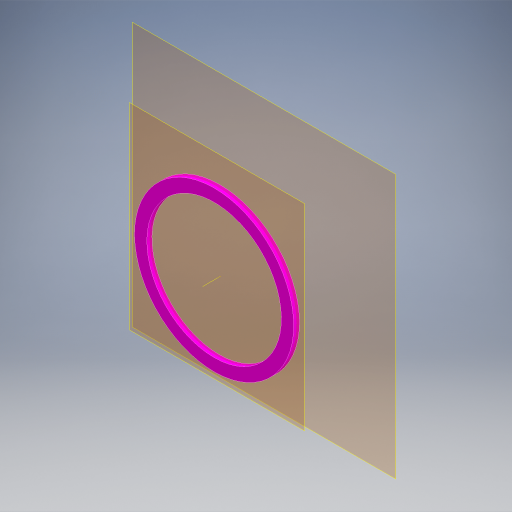
# Autodesk Inventor part: кольцо тсопов
Saved by Autodesk Inventor 2023 (Build 270158000, 158)
## iProperties
Created: 2025-03-03
Part Number: кольцо тсопов
Material: Типовые
Document SubType Name: Modeling
Designer: Ivan
Density: 1 g/cm^3
Appearance: Пурпурный
Author: Ivan
Autodesk Inventor part; units mm, degrees
ref_plane "YZ Plane" through (0, 0, 0) normal (1, 0, 0) x (0, 1, 0)
ref_plane "XZ Plane" through (0, 0, 0) normal (0, 1, 0) x (-1, 0, 0)
ref_plane "РабПлоскость1" through (0, 0, 0) normal (0, 0, 1) x (1, 0, 0)
sketch "Эскиз1" plane through (0, 0, 0) normal (0, 0, 1) x (1, 0, 0)
  circle A0 centre (-0.0031, 0.0005) radius 45.313 projected
  arc A1 (-32.0981, 35.7243) -> (-32.4617, 35.3942) centre (0, 0) ccw projected
  circle A2 centre (0, 0) radius 45.413
  circle A3 centre (0, 0) radius 48.0262
  point P0 (0, 0)
  point P1 (-32.4617, 35.3942)
  point P2 (-32.0981, 35.7243)
  dimension "d0" = 90.626
  dimension "d1" = 90.826
  constraints: 2 centre point, 2 coincident
  measures "d0" diameter of A0
  measures "d1" diameter of A2
ref_plane "РабПлоскость2" through (-45.3206, -45.317, 0.4115) normal (0, 0, 1) x (1, 0.0001, 0)
extrude "Выдавливание1" add sketch "Эскиз1" along normal blind 3.5 contours A3 A1
ref_plane "РабПлоскость3" through (0, 0, 1.75) normal (0, 0, 1) x (1, 0, 0)
sketch "Эскиз3" plane through (0, 0, 0) normal (0, 0, 1) x (1, 0, 0)
  arc A0 (-22.0856, 39.6831) -> (-7.3436, 35.1497) centre (-7.7664, 60.011) ccw projected
  line L0 (-7.3436, 35.1497) -> (7.3325, 35.1512) projected
  arc A1 (7.3325, 35.1512) -> (22.0736, 39.6875) centre (7.7504, 60.0125) ccw projected
  circle A2 centre (0, 0) radius 45.413 projected
  circle A3 centre (-15.1051, 31) radius 1.55 projected
  circle A4 centre (15.0949, 31.002) radius 1.55 projected
  arc A5 (-17.5837, 28.9218) -> (-32.0889, 32.1347) centre (-28.1894, 15.3907) ccw projected
  arc A6 (-16.8937, 28.4734) -> (-17.5837, 28.9218) centre (-22.6832, 20.3197) ccw projected
  arc A7 (-16.8937, 28.4734) -> (-9.3575, 28.0766) centre (-12.8523, 33.4648) ccw projected
  arc A8 (-5.0551, 30.151) -> (-5.054, 19.151) centre (-5.0545, 24.651) ccw projected
  line L1 (5.0449, 30.151) -> (-5.0551, 30.151) projected
  arc A9 (5.046, 19.151) -> (5.0449, 30.151) centre (5.0455, 24.651) ccw projected
  arc A10 (9.3461, 28.0795) -> (16.884, 28.4767) centre (12.8416, 33.4673) ccw projected
  arc A11 (17.5738, 28.9252) -> (16.884, 28.4767) centre (22.675, 20.3242) ccw projected
  arc A12 (32.0838, 32.1398) -> (17.5738, 28.9252) centre (28.1822, 15.3963) ccw projected
  point P0 (0, 0)
  point P1 (-22.0837, 39.6818)
extrude "Выдавливание2" [suppressed]
sketch "Эскиз4" plane through (0, 0, 0) normal (0, 0, -1) x (-1, 0, 0)
  circle A0 centre (-15.099, -31.001) radius 1.6 projected
  circle A1 centre (15.101, -31) radius 1.6 projected
  circle A2 centre (-15.101, 31) radius 1.6 projected
  circle A3 centre (15.099, 31.001) radius 1.6 projected
  arc A4 (47.464, 7.3269) -> (46.1696, 9.1429) centre (45.0118, 6.9484) ccw projected
  line L0 (46.1696, 9.1429) -> (46.154, 9.2214) projected
  arc A5 (46.154, 9.2214) -> (46.6549, 11.3945) centre (44.2445, 10.8058) ccw projected
  arc A6 (46.6549, 11.3945) -> (46.5359, 11.8709) centre (0, 0) ccw projected
  arc A7 (45.1226, 16.4459) -> (43.4988, 17.9745) centre (42.7913, 15.5962) ccw projected
  line L1 (43.4988, 17.9745) -> (43.4682, 18.0484) projected
  arc A8 (43.4682, 18.0484) -> (43.5355, 20.2775) centre (41.2862, 19.2298) ccw projected
  arc A9 (43.5355, 20.2775) -> (43.3259, 20.7215) centre (0, 0) ccw projected
  arc A10 (41.0471, 24.9329) -> (39.1563, 26.1153) centre (38.9264, 23.6447) ccw projected
  line L2 (39.1563, 26.1153) -> (39.1119, 26.1818) projected
  arc A11 (39.1119, 26.1818) -> (38.743, 28.3812) centre (36.7414, 26.9149) ccw projected
  arc A12 (38.743, 28.3812) -> (38.4508, 28.7758) centre (0, 0) ccw projected
  arc A13 (35.3942, 32.4617) -> (33.3091, 33.2525) centre (33.5656, 30.7846) ccw projected
  line L3 (33.3091, 33.2525) -> (33.2525, 33.3091) projected
  arc A14 (33.2525, 33.3091) -> (32.4617, 35.3942) centre (30.7846, 33.5656) ccw projected
  arc A15 (32.4617, 35.3942) -> (32.0981, 35.7243) centre (0, 0) ccw projected
  arc A16 (28.3812, 38.743) -> (26.1818, 39.1119) centre (26.9149, 36.7414) ccw projected
  line L4 (26.1818, 39.1119) -> (26.1153, 39.1563) projected
  arc A17 (26.1153, 39.1563) -> (24.9329, 41.0471) centre (23.6447, 38.9264) ccw projected
  arc A18 (24.9329, 41.0471) -> (24.5119, 41.2999) centre (0, 0) ccw projected
  arc A19 (20.2775, 43.5355) -> (18.0484, 43.4682) centre (19.2298, 41.2862) ccw projected
  line L5 (18.0484, 43.4682) -> (17.9745, 43.4988) projected
  arc A20 (17.9745, 43.4988) -> (16.4459, 45.1226) centre (15.5962, 42.7913) ccw projected
  arc A21 (16.4459, 45.1226) -> (15.9837, 45.2884) centre (0, 0) ccw projected
  arc A22 (11.3945, 46.6549) -> (9.2214, 46.154) centre (10.8058, 44.2445) ccw projected
  line L6 (9.2214, 46.154) -> (9.1429, 46.1696) projected
  arc A23 (9.1429, 46.1696) -> (7.3269, 47.464) centre (6.9484, 45.0118) ccw projected
  arc A24 (7.3269, 47.464) -> (6.8412, 47.5364) centre (0, 0) ccw projected
  arc A25 (2.0736, 47.9814) -> (0.04, 47.0662) centre (1.9665, 45.5024) ccw projected
  line L7 (0.04, 47.0662) -> (-0.04, 47.0662) projected
  arc A26 (-0.04, 47.0662) -> (-2.0736, 47.9814) centre (-1.9665, 45.5024) ccw projected
  arc A27 (-2.0736, 47.9814) -> (-2.5641, 47.9577) centre (0, 0) ccw projected
  arc A28 (-7.3269, 47.464) -> (-9.1429, 46.1696) centre (-6.9484, 45.0118) ccw projected
  line L8 (-9.1429, 46.1696) -> (-9.2214, 46.154) projected
  arc A29 (-9.2214, 46.154) -> (-11.3945, 46.6549) centre (-10.8058, 44.2445) ccw projected
  arc A30 (-11.3945, 46.6549) -> (-11.8709, 46.5359) centre (0, 0) ccw projected
  arc A31 (-16.4459, 45.1226) -> (-17.9745, 43.4988) centre (-15.5962, 42.7913) ccw projected
  line L9 (-17.9745, 43.4988) -> (-18.0484, 43.4682) projected
  arc A32 (-18.0484, 43.4682) -> (-20.2775, 43.5355) centre (-19.2298, 41.2862) ccw projected
  arc A33 (-20.2775, 43.5355) -> (-20.7215, 43.3259) centre (0, 0) ccw projected
  arc A34 (-24.9329, 41.0471) -> (-26.1153, 39.1563) centre (-23.6447, 38.9264) ccw projected
  line L10 (-26.1153, 39.1563) -> (-26.1818, 39.1119) projected
  arc A35 (-26.1818, 39.1119) -> (-28.3812, 38.743) centre (-26.9149, 36.7414) ccw projected
  arc A36 (-28.3812, 38.743) -> (-28.7758, 38.4508) centre (0, 0) ccw projected
  arc A37 (-32.4617, 35.3942) -> (-33.2525, 33.3091) centre (-30.7846, 33.5656) ccw projected
  line L11 (-33.2525, 33.3091) -> (-33.3091, 33.2525) projected
  arc A38 (-33.3091, 33.2525) -> (-35.3942, 32.4617) centre (-33.5656, 30.7846) ccw projected
  arc A39 (-35.3942, 32.4617) -> (-35.7243, 32.0981) centre (0, 0) ccw projected
  arc A40 (-38.743, 28.3812) -> (-39.1119, 26.1818) centre (-36.7414, 26.9149) ccw projected
  line L12 (-39.1119, 26.1818) -> (-39.1563, 26.1153) projected
  arc A41 (-39.1563, 26.1153) -> (-41.0471, 24.9329) centre (-38.9264, 23.6447) ccw projected
  arc A42 (-41.0471, 24.9329) -> (-41.2999, 24.5119) centre (0, 0) ccw projected
  arc A43 (-43.5355, 20.2775) -> (-43.4682, 18.0484) centre (-41.2862, 19.2298) ccw projected
  line L13 (-43.4682, 18.0484) -> (-43.4988, 17.9745) projected
  arc A44 (-43.4988, 17.9745) -> (-45.1226, 16.4459) centre (-42.7913, 15.5962) ccw projected
  arc A45 (-45.1226, 16.4459) -> (-45.2884, 15.9837) centre (0, 0) ccw projected
  arc A46 (-46.6549, 11.3945) -> (-46.154, 9.2214) centre (-44.2445, 10.8058) ccw projected
  line L14 (-46.154, 9.2214) -> (-46.1696, 9.1429) projected
  arc A47 (-46.1696, 9.1429) -> (-47.464, 7.3269) centre (-45.0118, 6.9484) ccw projected
  arc A48 (-47.464, 7.3269) -> (-47.5364, 6.8412) centre (0, 0) ccw projected
  arc A49 (-47.9814, 2.0736) -> (-47.0662, 0.04) centre (-45.5024, 1.9665) ccw projected
  line L15 (-47.0662, 0.04) -> (-47.0662, -0.04) projected
  arc A50 (-47.0662, -0.04) -> (-47.9814, -2.0736) centre (-45.5024, -1.9665) ccw projected
  arc A51 (-47.9814, -2.0736) -> (-47.9577, -2.5641) centre (0, 0) ccw projected
  arc A52 (-47.464, -7.3269) -> (-46.1696, -9.1429) centre (-45.0118, -6.9484) ccw projected
  line L16 (-46.1696, -9.1429) -> (-46.154, -9.2214) projected
  arc A53 (-46.154, -9.2214) -> (-46.6549, -11.3945) centre (-44.2445, -10.8058) ccw projected
  arc A54 (-46.6549, -11.3945) -> (-46.5359, -11.8709) centre (0, 0) ccw projected
  arc A55 (-45.1226, -16.4459) -> (-43.4988, -17.9745) centre (-42.7913, -15.5962) ccw projected
  line L17 (-43.4988, -17.9745) -> (-43.4682, -18.0484) projected
  arc A56 (-43.4682, -18.0484) -> (-43.5355, -20.2775) centre (-41.2862, -19.2298) ccw projected
  arc A57 (-43.5355, -20.2775) -> (-43.3259, -20.7215) centre (0, 0) ccw projected
  arc A58 (-41.0471, -24.9329) -> (-39.1563, -26.1153) centre (-38.9264, -23.6447) ccw projected
  line L18 (-39.1563, -26.1153) -> (-39.1119, -26.1818) projected
  arc A59 (-39.1119, -26.1818) -> (-38.743, -28.3812) centre (-36.7414, -26.9149) ccw projected
  arc A60 (-38.743, -28.3812) -> (-38.4508, -28.7758) centre (0, 0) ccw projected
  arc A61 (-35.3942, -32.4617) -> (-33.3091, -33.2525) centre (-33.5656, -30.7846) ccw projected
  line L19 (-33.3091, -33.2525) -> (-33.2525, -33.3091) projected
  arc A62 (-33.2525, -33.3091) -> (-32.4617, -35.3942) centre (-30.7846, -33.5656) ccw projected
  arc A63 (-32.4617, -35.3942) -> (-32.0981, -35.7243) centre (0, 0) ccw projected
  arc A64 (-28.3812, -38.743) -> (-26.1818, -39.1119) centre (-26.9149, -36.7414) ccw projected
  line L20 (-26.1818, -39.1119) -> (-26.1153, -39.1563) projected
  arc A65 (-26.1153, -39.1563) -> (-24.9329, -41.0471) centre (-23.6447, -38.9264) ccw projected
  arc A66 (-24.9329, -41.0471) -> (-24.5119, -41.2999) centre (0, 0) ccw projected
  arc A67 (-20.2775, -43.5355) -> (-18.0484, -43.4682) centre (-19.2298, -41.2862) ccw projected
  line L21 (-18.0484, -43.4682) -> (-17.9745, -43.4988) projected
  arc A68 (-17.9745, -43.4988) -> (-16.4459, -45.1226) centre (-15.5962, -42.7913) ccw projected
  arc A69 (-16.4459, -45.1226) -> (-15.9837, -45.2884) centre (0, 0) ccw projected
  arc A70 (-11.3945, -46.6549) -> (-9.2214, -46.154) centre (-10.8058, -44.2445) ccw projected
  line L22 (-9.2214, -46.154) -> (-9.1429, -46.1696) projected
  arc A71 (-9.1429, -46.1696) -> (-7.3269, -47.464) centre (-6.9484, -45.0118) ccw projected
  arc A72 (-7.3269, -47.464) -> (-6.8412, -47.5364) centre (0, 0) ccw projected
  arc A73 (-2.0736, -47.9814) -> (-0.04, -47.0662) centre (-1.9665, -45.5024) ccw projected
  line L23 (-0.04, -47.0662) -> (0.04, -47.0662) projected
  arc A74 (0.04, -47.0662) -> (2.0736, -47.9814) centre (1.9665, -45.5024) ccw projected
  arc A75 (2.0736, -47.9814) -> (2.5641, -47.9577) centre (0, 0) ccw projected
  arc A76 (7.3269, -47.464) -> (9.1429, -46.1696) centre (6.9484, -45.0118) ccw projected
  line L24 (9.1429, -46.1696) -> (9.2214, -46.154) projected
  arc A77 (9.2214, -46.154) -> (11.3945, -46.6549) centre (10.8058, -44.2445) ccw projected
  arc A78 (11.3945, -46.6549) -> (11.8709, -46.5359) centre (0, 0) ccw projected
  arc A79 (16.4459, -45.1226) -> (17.9745, -43.4988) centre (15.5962, -42.7913) ccw projected
  line L25 (17.9745, -43.4988) -> (18.0484, -43.4682) projected
  arc A80 (18.0484, -43.4682) -> (20.2775, -43.5355) centre (19.2298, -41.2862) ccw projected
  arc A81 (20.2775, -43.5355) -> (20.7215, -43.3259) centre (0, 0) ccw projected
  arc A82 (24.9329, -41.0471) -> (26.1153, -39.1563) centre (23.6447, -38.9264) ccw projected
  line L26 (26.1153, -39.1563) -> (26.1818, -39.1119) projected
  arc A83 (26.1818, -39.1119) -> (28.3812, -38.743) centre (26.9149, -36.7414) ccw projected
  arc A84 (28.3812, -38.743) -> (28.7758, -38.4508) centre (0, 0) ccw projected
  arc A85 (32.4617, -35.3942) -> (33.2525, -33.3091) centre (30.7846, -33.5656) ccw projected
  line L27 (33.2525, -33.3091) -> (33.3091, -33.2525) projected
  arc A86 (33.3091, -33.2525) -> (35.3942, -32.4617) centre (33.5656, -30.7846) ccw projected
  arc A87 (35.3942, -32.4617) -> (35.7243, -32.0981) centre (0, 0) ccw projected
  arc A88 (38.743, -28.3812) -> (39.1119, -26.1818) centre (36.7414, -26.9149) ccw projected
  line L28 (39.1119, -26.1818) -> (39.1563, -26.1153) projected
  arc A89 (39.1563, -26.1153) -> (41.0471, -24.9329) centre (38.9264, -23.6447) ccw projected
  arc A90 (41.0471, -24.9329) -> (41.2999, -24.5119) centre (0, 0) ccw projected
  arc A91 (43.5355, -20.2775) -> (43.4682, -18.0484) centre (41.2862, -19.2298) ccw projected
  line L29 (43.4682, -18.0484) -> (43.4988, -17.9745) projected
  arc A92 (43.4988, -17.9745) -> (45.1226, -16.4459) centre (42.7913, -15.5962) ccw projected
  arc A93 (45.1226, -16.4459) -> (45.2884, -15.9837) centre (0, 0) ccw projected
  arc A94 (46.6549, -11.3945) -> (46.154, -9.2214) centre (44.2445, -10.8058) ccw projected
  line L30 (46.154, -9.2214) -> (46.1696, -9.1429) projected
  arc A95 (46.1696, -9.1429) -> (47.464, -7.3269) centre (45.0118, -6.9484) ccw projected
  arc A96 (47.464, -7.3269) -> (47.5364, -6.8412) centre (0, 0) ccw projected
  arc A97 (47.9814, -2.0736) -> (47.0662, -0.04) centre (45.5024, -1.9665) ccw projected
  line L31 (47.0662, -0.04) -> (47.0662, 0.04) projected
  arc A98 (47.0662, 0.04) -> (47.9814, 2.0736) centre (45.5024, 1.9665) ccw projected
  arc A99 (47.9814, 2.0736) -> (47.9577, 2.5641) centre (0, 0) ccw projected
  arc A100 (27.9976, -29.0215) -> (27.9957, 29.0233) centre (0, 0) ccw projected
  arc A101 (22.6601, -30.3182) -> (27.9976, -29.0215) centre (22.6882, -18.8005) ccw projected
  arc A102 (16.8956, -28.4723) -> (22.6601, -30.3182) centre (22.6845, -20.3182) ccw projected
  arc A103 (16.8956, -28.4723) -> (12.0606, -31.6048) centre (15.101, -31) ccw projected
  arc A104 (5.6683, -39.9247) -> (12.0606, -31.6048) centre (4.6141, -32.4992) ccw projected
  arc A105 (-5.6658, -39.9251) -> (5.6683, -39.9247) centre (0, 0) ccw projected
  arc A106 (-12.0585, -31.6056) -> (-5.6658, -39.9251) centre (-4.612, -32.4995) ccw projected
  arc A107 (-12.0585, -31.6056) -> (-16.8937, -28.4734) centre (-15.099, -31.001) ccw projected
  arc A108 (-22.6581, -30.3197) -> (-16.8937, -28.4734) centre (-22.6832, -20.3197) ccw projected
  arc A109 (-27.9957, -29.0233) -> (-22.6581, -30.3197) centre (-22.687, -18.802) ccw projected
  arc A110 (-27.9976, 29.0215) -> (-27.9957, -29.0233) centre (0, 0) ccw projected
  arc A111 (-22.6601, 30.3182) -> (-27.9976, 29.0215) centre (-22.6882, 18.8005) ccw projected
  arc A112 (-16.8956, 28.4723) -> (-22.6601, 30.3182) centre (-22.6845, 20.3182) ccw projected
  arc A113 (-16.8956, 28.4723) -> (-12.0606, 31.6048) centre (-15.101, 31) ccw projected
  arc A114 (-5.6683, 39.9247) -> (-12.0606, 31.6048) centre (-4.6141, 32.4992) ccw projected
  arc A115 (5.6658, 39.9251) -> (-5.6683, 39.9247) centre (0, 0) ccw projected
  arc A116 (12.0585, 31.6056) -> (5.6658, 39.9251) centre (4.612, 32.4995) ccw projected
  arc A117 (12.0585, 31.6056) -> (16.8937, 28.4734) centre (15.099, 31.001) ccw projected
  arc A118 (22.6581, 30.3197) -> (16.8937, 28.4734) centre (22.6832, 20.3197) ccw projected
  arc A119 (27.9957, 29.0233) -> (22.6581, 30.3197) centre (22.687, 18.802) ccw projected
  circle A120 centre (0, 0) radius 48.0262 projected
  circle A121 centre (0, 0) radius 47.4785
  arc A122 (46.6623, -10.2485) -> (46.1696, -9.2404) centre (44.2445, -10.8058) ccw
  arc A123 (-3.4564, -47.5061) -> (-2.5641, -47.9577) centre (-2.4979, -46.7194) ccw projected
  arc A124 (-2.5641, -47.9577) -> (-2.0736, -47.9814) centre (0, 0) ccw projected
  arc A125 (2.5641, -47.9577) -> (3.4564, -47.5061) centre (2.4979, -46.7194) ccw projected
  line L32 (3.4564, -47.5061) -> (4.5479, -46.1761) projected
  line L33 (4.5479, -46.1761) -> (5.878, -47.2676) projected
  arc A126 (5.878, -47.2676) -> (6.8412, -47.5364) centre (6.6646, -46.3091) ccw projected
  arc A127 (6.8412, -47.5364) -> (7.3269, -47.464) centre (0, 0) ccw projected
  arc A128 (11.8709, -46.5359) -> (12.658, -45.9189) centre (11.5644, -45.3344) ccw projected
  line L34 (12.658, -45.9189) -> (13.4691, -44.4016) projected
  line L35 (13.4691, -44.4016) -> (14.9865, -45.2126) projected
  arc A129 (14.9865, -45.2126) -> (15.9837, -45.2884) centre (15.571, -44.119) ccw projected
  arc A130 (15.9837, -45.2884) -> (16.4459, -45.1226) centre (0, 0) ccw projected
  arc A131 (20.7215, -43.3259) -> (21.3731, -42.5672) centre (20.1865, -42.2072) ccw projected
  line L36 (21.3731, -42.5672) -> (21.8726, -40.9207) projected
  line L37 (21.8726, -40.9207) -> (23.519, -41.4202) projected
  arc A132 (23.519, -41.4202) -> (24.5119, -41.2999) centre (23.879, -40.2336) ccw projected
  arc A133 (24.5119, -41.2999) -> (24.9329, -41.0471) centre (0, 0) ccw projected
  arc A134 (28.7758, -38.4508) -> (29.2669, -37.5796) centre (28.0329, -37.458) ccw projected
  line L38 (29.2669, -37.5796) -> (29.4355, -35.8673) projected
  line L39 (29.4355, -35.8673) -> (31.1478, -36.0359) projected
  arc A135 (31.1478, -36.0359) -> (32.0981, -35.7243) centre (31.2693, -34.8019) ccw projected
  arc A136 (32.0981, -35.7243) -> (32.4617, -35.3942) centre (0, 0) ccw projected
  arc A137 (35.7243, -32.0981) -> (36.0359, -31.1478) centre (34.8019, -31.2693) ccw projected
  line L40 (36.0359, -31.1478) -> (35.8673, -29.4355) projected
  line L41 (35.8673, -29.4355) -> (37.5796, -29.2669) projected
  arc A138 (37.5796, -29.2669) -> (38.4508, -28.7758) centre (37.458, -28.0329) ccw projected
  arc A139 (38.4508, -28.7758) -> (38.743, -28.3812) centre (0, 0) ccw projected
  arc A140 (41.2999, -24.5119) -> (41.4202, -23.519) centre (40.2336, -23.879) ccw projected
  line L42 (41.4202, -23.519) -> (40.9207, -21.8726) projected
  line L43 (40.9207, -21.8726) -> (42.5672, -21.3731) projected
  arc A141 (42.5672, -21.3731) -> (43.3259, -20.7215) centre (42.2072, -20.1865) ccw projected
  arc A142 (43.3259, -20.7215) -> (43.5355, -20.2775) centre (0, 0) ccw projected
  arc A143 (45.2884, -15.9837) -> (45.2126, -14.9865) centre (44.119, -15.571) ccw projected
  line L44 (45.2126, -14.9865) -> (44.4016, -13.4691) projected
  line L45 (44.4016, -13.4691) -> (45.9189, -12.658) projected
  arc A144 (45.9189, -12.658) -> (46.5359, -11.8709) centre (45.3344, -11.5644) ccw projected
  arc A145 (46.5359, -11.8709) -> (46.6549, -11.3945) centre (0, 0) ccw projected
  arc A146 (47.5364, -6.8412) -> (47.2676, -5.878) centre (46.3091, -6.6646) ccw projected
  line L46 (47.2676, -5.878) -> (46.1761, -4.5479) projected
  line L47 (46.1761, -4.5479) -> (47.5061, -3.4564) projected
  arc A147 (47.5061, -3.4564) -> (47.9577, -2.5641) centre (46.7194, -2.4979) ccw projected
  arc A148 (47.9577, -2.5641) -> (47.9814, -2.0736) centre (0, 0) ccw projected
  arc A149 (47.9577, 2.5641) -> (47.5061, 3.4564) centre (46.7194, 2.4979) ccw projected
  line L48 (47.5061, 3.4564) -> (46.1761, 4.5479) projected
  line L49 (46.1761, 4.5479) -> (47.2676, 5.878) projected
  arc A150 (47.2676, 5.878) -> (47.5364, 6.8412) centre (46.3091, 6.6646) ccw projected
  arc A151 (47.5364, 6.8412) -> (47.464, 7.3269) centre (0, 0) ccw projected
  arc A152 (46.5359, 11.8709) -> (45.9189, 12.658) centre (45.3344, 11.5644) ccw projected
  line L50 (45.9189, 12.658) -> (44.4016, 13.4691) projected
  line L51 (44.4016, 13.4691) -> (45.2126, 14.9865) projected
  arc A153 (45.2126, 14.9865) -> (45.2884, 15.9837) centre (44.119, 15.571) ccw projected
  arc A154 (45.2884, 15.9837) -> (45.1226, 16.4459) centre (0, 0) ccw projected
  arc A155 (43.3259, 20.7215) -> (42.5672, 21.3731) centre (42.2072, 20.1865) ccw projected
  line L52 (42.5672, 21.3731) -> (40.9207, 21.8726) projected
  line L53 (40.9207, 21.8726) -> (41.4202, 23.519) projected
  arc A156 (41.4202, 23.519) -> (41.2999, 24.5119) centre (40.2336, 23.879) ccw projected
  arc A157 (41.2999, 24.5119) -> (41.0471, 24.9329) centre (0, 0) ccw projected
  arc A158 (38.4508, 28.7758) -> (37.5796, 29.2669) centre (37.458, 28.0329) ccw projected
  line L54 (37.5796, 29.2669) -> (35.8673, 29.4355) projected
  line L55 (35.8673, 29.4355) -> (36.0359, 31.1478) projected
  arc A159 (36.0359, 31.1478) -> (35.7243, 32.0981) centre (34.8019, 31.2693) ccw projected
  arc A160 (35.7243, 32.0981) -> (35.3942, 32.4617) centre (0, 0) ccw projected
  arc A161 (32.0981, 35.7243) -> (31.1478, 36.0359) centre (31.2693, 34.8019) ccw projected
  line L56 (31.1478, 36.0359) -> (29.4355, 35.8673) projected
  line L57 (29.4355, 35.8673) -> (29.2669, 37.5796) projected
  arc A162 (29.2669, 37.5796) -> (28.7758, 38.4508) centre (28.0329, 37.458) ccw projected
  arc A163 (28.7758, 38.4508) -> (28.3812, 38.743) centre (0, 0) ccw projected
  arc A164 (24.5119, 41.2999) -> (23.519, 41.4202) centre (23.879, 40.2336) ccw projected
  line L58 (23.519, 41.4202) -> (21.8726, 40.9207) projected
  line L59 (21.8726, 40.9207) -> (21.3731, 42.5672) projected
  arc A165 (21.3731, 42.5672) -> (20.7215, 43.3259) centre (20.1865, 42.2072) ccw projected
  arc A166 (20.7215, 43.3259) -> (20.2775, 43.5355) centre (0, 0) ccw projected
  arc A167 (15.9837, 45.2884) -> (14.9865, 45.2126) centre (15.571, 44.119) ccw projected
  line L60 (14.9865, 45.2126) -> (13.4691, 44.4016) projected
  line L61 (13.4691, 44.4016) -> (12.658, 45.9189) projected
  arc A168 (12.658, 45.9189) -> (11.8709, 46.5359) centre (11.5644, 45.3344) ccw projected
  arc A169 (11.8709, 46.5359) -> (11.3945, 46.6549) centre (0, 0) ccw projected
  arc A170 (6.8412, 47.5364) -> (5.878, 47.2676) centre (6.6646, 46.3091) ccw projected
  line L62 (5.878, 47.2676) -> (4.5479, 46.1761) projected
  line L63 (4.5479, 46.1761) -> (3.4564, 47.5061) projected
  arc A171 (3.4564, 47.5061) -> (2.5641, 47.9577) centre (2.4979, 46.7194) ccw projected
  arc A172 (2.5641, 47.9577) -> (2.0736, 47.9814) centre (0, 0) ccw projected
  arc A173 (-2.5641, 47.9577) -> (-3.4564, 47.5061) centre (-2.4979, 46.7194) ccw projected
  line L64 (-3.4564, 47.5061) -> (-4.5479, 46.1761) projected
  line L65 (-4.5479, 46.1761) -> (-5.878, 47.2676) projected
  arc A174 (-5.878, 47.2676) -> (-6.8412, 47.5364) centre (-6.6646, 46.3091) ccw projected
  arc A175 (-6.8412, 47.5364) -> (-7.3269, 47.464) centre (0, 0) ccw projected
  arc A176 (-11.8709, 46.5359) -> (-12.658, 45.9189) centre (-11.5644, 45.3344) ccw projected
  line L66 (-12.658, 45.9189) -> (-13.4691, 44.4016) projected
  line L67 (-13.4691, 44.4016) -> (-14.9865, 45.2126) projected
  arc A177 (-14.9865, 45.2126) -> (-15.9837, 45.2884) centre (-15.571, 44.119) ccw projected
  arc A178 (-15.9837, 45.2884) -> (-16.4459, 45.1226) centre (0, 0) ccw projected
  arc A179 (-20.7215, 43.3259) -> (-21.3731, 42.5672) centre (-20.1865, 42.2072) ccw projected
  line L68 (-21.3731, 42.5672) -> (-21.8726, 40.9207) projected
  line L69 (-21.8726, 40.9207) -> (-23.519, 41.4202) projected
  arc A180 (-23.519, 41.4202) -> (-24.5119, 41.2999) centre (-23.879, 40.2336) ccw projected
  arc A181 (-24.5119, 41.2999) -> (-24.9329, 41.0471) centre (0, 0) ccw projected
  arc A182 (-28.7758, 38.4508) -> (-29.2669, 37.5796) centre (-28.0329, 37.458) ccw projected
  line L70 (-29.2669, 37.5796) -> (-29.4355, 35.8673) projected
  line L71 (-29.4355, 35.8673) -> (-31.1478, 36.0359) projected
  arc A183 (-31.1478, 36.0359) -> (-32.0981, 35.7243) centre (-31.2693, 34.8019) ccw projected
  arc A184 (-32.0981, 35.7243) -> (-32.4617, 35.3942) centre (0, 0) ccw projected
  arc A185 (-35.7243, 32.0981) -> (-36.0359, 31.1478) centre (-34.8019, 31.2693) ccw projected
  line L72 (-36.0359, 31.1478) -> (-35.8673, 29.4355) projected
  line L73 (-35.8673, 29.4355) -> (-37.5796, 29.2669) projected
  arc A186 (-37.5796, 29.2669) -> (-38.4508, 28.7758) centre (-37.458, 28.0329) ccw projected
  arc A187 (-38.4508, 28.7758) -> (-38.743, 28.3812) centre (0, 0) ccw projected
  arc A188 (-41.2999, 24.5119) -> (-41.4202, 23.519) centre (-40.2336, 23.879) ccw projected
  line L74 (-41.4202, 23.519) -> (-40.9207, 21.8726) projected
  line L75 (-40.9207, 21.8726) -> (-42.5672, 21.3731) projected
  arc A189 (-42.5672, 21.3731) -> (-43.3259, 20.7215) centre (-42.2072, 20.1865) ccw projected
  arc A190 (-43.3259, 20.7215) -> (-43.5355, 20.2775) centre (0, 0) ccw projected
  arc A191 (-45.2884, 15.9837) -> (-45.2126, 14.9865) centre (-44.119, 15.571) ccw projected
  line L76 (-45.2126, 14.9865) -> (-44.4016, 13.4691) projected
  line L77 (-44.4016, 13.4691) -> (-45.9189, 12.658) projected
  arc A192 (-45.9189, 12.658) -> (-46.5359, 11.8709) centre (-45.3344, 11.5644) ccw projected
  arc A193 (-46.5359, 11.8709) -> (-46.6549, 11.3945) centre (0, 0) ccw projected
  arc A194 (-47.5364, 6.8412) -> (-47.2676, 5.878) centre (-46.3091, 6.6646) ccw projected
  line L78 (-47.2676, 5.878) -> (-46.1761, 4.5479) projected
  line L79 (-46.1761, 4.5479) -> (-47.5061, 3.4564) projected
  arc A195 (-47.5061, 3.4564) -> (-47.9577, 2.5641) centre (-46.7194, 2.4979) ccw projected
  arc A196 (-47.9577, 2.5641) -> (-47.9814, 2.0736) centre (0, 0) ccw projected
  arc A197 (-47.9577, -2.5641) -> (-47.5061, -3.4564) centre (-46.7194, -2.4979) ccw projected
  line L80 (-47.5061, -3.4564) -> (-46.1761, -4.5479) projected
  line L81 (-46.1761, -4.5479) -> (-47.2676, -5.878) projected
  arc A198 (-47.2676, -5.878) -> (-47.5364, -6.8412) centre (-46.3091, -6.6646) ccw projected
  arc A199 (-47.5364, -6.8412) -> (-47.464, -7.3269) centre (0, 0) ccw projected
  arc A200 (-46.5359, -11.8709) -> (-45.9189, -12.658) centre (-45.3344, -11.5644) ccw projected
  line L82 (-45.9189, -12.658) -> (-44.4016, -13.4691) projected
  line L83 (-44.4016, -13.4691) -> (-45.2126, -14.9865) projected
  arc A201 (-45.2126, -14.9865) -> (-45.2884, -15.9837) centre (-44.119, -15.571) ccw projected
  arc A202 (-45.2884, -15.9837) -> (-45.1226, -16.4459) centre (0, 0) ccw projected
  arc A203 (-43.3259, -20.7215) -> (-42.5672, -21.3731) centre (-42.2072, -20.1865) ccw projected
  line L84 (-42.5672, -21.3731) -> (-40.9207, -21.8726) projected
  line L85 (-40.9207, -21.8726) -> (-41.4202, -23.519) projected
  arc A204 (-41.4202, -23.519) -> (-41.2999, -24.5119) centre (-40.2336, -23.879) ccw projected
  arc A205 (-41.2999, -24.5119) -> (-41.0471, -24.9329) centre (0, 0) ccw projected
  arc A206 (-38.4508, -28.7758) -> (-37.5796, -29.2669) centre (-37.458, -28.0329) ccw projected
  line L86 (-37.5796, -29.2669) -> (-35.8673, -29.4355) projected
  line L87 (-35.8673, -29.4355) -> (-36.0359, -31.1478) projected
  arc A207 (-36.0359, -31.1478) -> (-35.7243, -32.0981) centre (-34.8019, -31.2693) ccw projected
  arc A208 (-35.7243, -32.0981) -> (-35.3942, -32.4617) centre (0, 0) ccw projected
  arc A209 (-32.0981, -35.7243) -> (-31.1478, -36.0359) centre (-31.2693, -34.8019) ccw projected
  line L88 (-31.1478, -36.0359) -> (-29.4355, -35.8673) projected
  line L89 (-29.4355, -35.8673) -> (-29.2669, -37.5796) projected
  arc A210 (-29.2669, -37.5796) -> (-28.7758, -38.4508) centre (-28.0329, -37.458) ccw projected
  arc A211 (-28.7758, -38.4508) -> (-28.3812, -38.743) centre (0, 0) ccw projected
  arc A212 (-24.5119, -41.2999) -> (-23.519, -41.4202) centre (-23.879, -40.2336) ccw projected
  line L90 (-23.519, -41.4202) -> (-21.8726, -40.9207) projected
  line L91 (-21.8726, -40.9207) -> (-21.3731, -42.5672) projected
  arc A213 (-21.3731, -42.5672) -> (-20.7215, -43.3259) centre (-20.1865, -42.2072) ccw projected
  arc A214 (-20.7215, -43.3259) -> (-20.2775, -43.5355) centre (0, 0) ccw projected
  arc A215 (-15.9837, -45.2884) -> (-14.9865, -45.2126) centre (-15.571, -44.119) ccw projected
  line L92 (-14.9865, -45.2126) -> (-13.4691, -44.4016) projected
  line L93 (-13.4691, -44.4016) -> (-12.658, -45.9189) projected
  arc A216 (-12.658, -45.9189) -> (-11.8709, -46.5359) centre (-11.5644, -45.3344) ccw projected
  arc A217 (-11.8709, -46.5359) -> (-11.3945, -46.6549) centre (0, 0) ccw projected
  arc A218 (-6.8412, -47.5364) -> (-5.878, -47.2676) centre (-6.6646, -46.3091) ccw projected
  line L94 (-5.878, -47.2676) -> (-4.5479, -46.1761) projected
  line L95 (-4.5479, -46.1761) -> (-3.4564, -47.5061) projected
  point P0 (0, 0)
  point P1 (46.4737, -9.7162)
  constraints: 5 point on circle, 1 centre point, 1 coincident, 1 concentric, 4 other
sketch "Эскиз5" plane through (0, 0, 0) normal (0, 0, -1) x (-1, 0, 0)
  line L0 (4.5479, -46.1761) -> (0, 0) construction
  circle A0 centre (0, 0) radius 48.0262 projected
  arc A1 (3.1624, -47.9219) -> (6.2475, -47.6181) centre (0, 0) ccw
  line L1 (6.2475, -47.6181) -> (4.553, -46.2275)
  line L2 (4.553, -46.2275) -> (3.1624, -47.9219)
  line L3 (6.2475, -47.6181) -> (6.1901, -47.0353)
  dimension "d7" = 45
  dimension "d8" = 45
  dimension "d9" = 3.1
  constraints: 8 end point, 4 point on circle, 1 centre point, 1 coincident, 1 perpendicular, 1 point on line, 1 other
  measures "d7" angle of L2 L0
  measures "d8" angle of L1 L3
  measures "d9" distance from line of L2.end L3
extrude "Выдавливание3" [suppressed]
sketch "Эскиз6" plane through (0, 0, -13.2) normal (0, 0, -1) x (-1, 0, 0)
  arc A0 (3.1624, -47.9219) -> (6.2475, -47.6181) centre (0, 0) ccw projected
  line L0 (6.2475, -47.6181) -> (4.553, -46.2275) projected
  line L1 (4.553, -46.2275) -> (3.1624, -47.9219) projected
  line L2 (3.1624, -47.9219) -> (4.308, -43.7395)
  line L3 (4.308, -43.7395) -> (6.2475, -47.6181)
  circle A1 centre (0, 0) radius 48.0262 projected
  line L4 (4.7074, -47.7949) -> (4.553, -46.2275)
  line L5 (4.553, -46.2275) -> (4.5494, -46.2278)
  point P0 (0, 0)
  dimension "d12" = 2.5
  constraints: 8 end point, 2 point on circle, 1 perpendicular, 1 point on line
  measures "d12" distance from line of L2.end L5
extrude "Выдавливание4" [suppressed]
chamfer "Фаска1" [suppressed]
pattern_circular "Круговой массив1" [suppressed]
sketch "Эскиз8" plane through (0, 0, 0) normal (1, 0, 0) x (0, 1, 0)
  line L0 (-45.413, 3.5) -> (45.413, 3.5) projected
  line L1 (-45.413, 0) -> (45.413, 0) projected
  line L2 (-45.3125, 0.4115) -> (45.3135, 0.4115) projected
  line L3 (-45.3125, 0) -> (45.3135, 0) projected
  line L4 (-42.7497, 2.1915) -> (-43.2497, 2.1915) projected
  line L5 (-45.413, 3.5) -> (45.413, 3.5) projected
  line L6 (-42.7498, 2.1915) -> (-42.7498, -0.7) projected
  line L7 (-45.413, 3.5) -> (-45.413, 0) projected
  line L8 (-45.413, 2.6) -> (-43.6924, 2.6)
  line L9 (-43.6924, 2.6) -> (-43.6924, 3.5) construction
  line L10 (48.0262, 3.5) -> (-48.0262, 3.5) projected
  line L11 (-45.3125, 0.4215) -> (-38.3644, 0.4215)
  arc A0 (-41.5139, 0.4215) -> (-43.6924, 2.6) centre (-43.6924, 0.4215) ccw
  line L12 (-41.5139, 0.4215) -> (-41.5139, 1.7216)
  arc A1 (-40.6139, 0.4215) -> (-43.6924, 3.5) centre (-43.6924, 0.4215) ccw construction
  line L13 (-40.6139, 0.4215) -> (-40.6139, 0.1377)
  line L14 (0, -1.6613) -> (0, 5.0678) projected
  line L15 (-40.6139, 0.4215) -> (-40.6139, 3.5)
  line L16 (-40.6139, 3.5) -> (-43.6924, 3.5)
  point P0 (0, 0)
  dimension "d21" = 0.01
  dimension "d22" = 3.8991
  dimension "d23" = 0.9
  dimension "d24" = 0.9
  constraints: 14 end point, 6 point on line, 4 point on circle, 4 tangent, 2 centre point, 2 horizontal, 2 perpendicular, 2 vertical, 1 collinear
  measures "d21" distance between parallel lines of L2 L11
  measures "d22" distance between parallel lines of L7 L12
  measures "d23" distance of L9.end L8.end
  measures "d24" distance of L13.start L12.start
revolve "Вращение1" add sketch "Эскиз8" angle 360 about axis through (0, 0, 0) along (0, 0, 1) contours L0 L15 L11 A0 L8 L7
